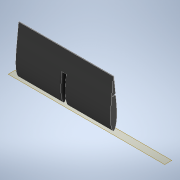
# Autodesk Inventor part: IISRD_Horizontal_tail_Control_surface
Saved by Autodesk Inventor 2021 (Build 250183000, 183)
## iProperties
Created: 2020-10-19
Part Number: IISRD_Horizontal_tail_Control_surface
Material: EPP Foam
Document SubType Name: Modeling
Designer: Kanenas
Mass: 7.28313 g
Surface Area: 775.374 cm^2
Volume: 364.157 cm^3
Density: 0.02 g/cm^3
Appearance: Generic
Author: Kanenas
Autodesk Inventor part; units mm, degrees
ref_plane "YZ Plane" through (0, 0, 0) normal (1, 0, 0) x (0, 1, 0)
sketch "Sketch1" plane through (0, 0, 0) normal (1, 0, 0) x (0, 1, 0)
  spline S0 degree 5 poles (140, 0) (140, 0.008) (139.6909, 0.023) (138.2456, 0.0648) (138.0851, 0.2448) (134.3445, 0.4509) (132.587, 0.7525) (128.0169, 1.03) (124.0758, 1.4239) (118.6617, 1.8648) (113.1342, 2.4056) (106.871, 3.0117) (100.3305, 3.6855) (93.4209, 4.4087) (86.3255, 5.1563) (79.0958, 5.9053) (71.8372, 6.629) (64.6288, 7.2884) (57.549, 7.8613) (50.671, 8.3132) (44.0585, 8.6184) (37.7676, 8.751) (31.8409, 8.7076) (26.336, 8.4735) (21.2773, 8.0467) (16.7064, 7.4272) (12.6313, 6.6359) (9.1041, 5.7147) (6.0909, 4.6974) (3.705, 3.6163) (1.758, 2.4782) (0.495, 1.2916) (-0.4137, 0) (0.495, -1.2916) (1.758, -2.4782) (3.705, -3.6163) (6.0909, -4.6974) (9.1041, -5.7147) (12.6313, -6.6359) (16.7064, -7.4272) (21.2773, -8.0467) (26.336, -8.4735) (31.8409, -8.7076) (37.7676, -8.751) (44.0585, -8.6184) (50.671, -8.3132) (57.549, -7.8613) (64.6288, -7.2884) (71.8372, -6.629) (79.0958, -5.9053) (86.3255, -5.1563) (93.4209, -4.4087) (100.3305, -3.6855) (106.871, -3.0117) (113.1342, -2.4056) (118.6617, -1.8648) (124.0758, -1.4239) (128.0169, -1.03) (132.587, -0.7525) (134.3445, -0.4509) (138.0851, -0.2448) (138.2456, -0.0648) (139.6909, -0.023) (140, -0.008) (140, 0) knots 0 0 0 0 0 0 0.009495 0.017637 0.028865 0.042353 0.057559 0.074188 0.092027 0.110874 0.13054 0.150849 0.171639 0.192755 0.214053 0.235397 0.256657 0.277714 0.298457 0.318784 0.338597 0.357809 0.37634 0.394116 0.411062 0.427101 0.442142 0.456085 0.468809 0.480163 0.490364 0.5 0.509636 0.519837 0.531191 0.543915 0.557858 0.572899 0.588938 0.605884 0.62366 0.642191 0.661403 0.681216 0.701543 0.722286 0.743343 0.764603 0.785947 0.807245 0.828361 0.849151 0.86946 0.889126 0.907973 0.925812 0.942441 0.957647 0.971135 0.982363 0.990505 1 1 1 1 1 1
  line L0 (130, 16.3724) -> (164.1986, 16.3724)
  line L1 (164.1986, 16.3724) -> (164.1986, -9.4783)
  line L2 (164.1986, -9.4783) -> (130, -9.4783)
  line L3 (130, -9.4783) -> (130, 16.3724)
  line L4 (37.4346, 8.7094) -> (37.4346, -8.7094) construction
  line L5 (20.881, 23.052) -> (20.881, -17.073) construction
  line L6 (57.3608, 24.3842) -> (57.3608, -18.5196) construction
  line L7 (20.881, -17.073) -> (57.3608, -17.073) construction
  line L8 (39.1209, -17.073) -> (39.1209, 13.7303) construction
  point P0 (138.0834, 0.1512)
  point P1 (135.8252, 0.3794)
  point P2 (132.797, 0.6664)
  point P3 (129.0044, 0.9884)
  point P4 (124.4796, 1.3706)
  point P5 (119.294, 1.8284)
  point P6 (113.526, 2.3674)
  point P7 (107.2624, 2.982)
  point P8 (100.5956, 3.661)
  point P9 (93.6194, 4.389)
  point P10 (86.4304, 5.1422)
  point P11 (79.1224, 5.8954)
  point P12 (71.785, 6.6192)
  point P13 (64.505, 7.28)
  point P14 (57.3608, 7.8484)
  point P15 (50.4266, 8.2936)
  point P16 (43.7668, 8.5876)
  point P17 (31.479, 8.6478)
  point P18 (25.9504, 8.393)
  point P19 (20.881, 7.9408)
  point P20 (16.2974, 7.2954)
  point P21 (12.222, 6.4778)
  point P22 (8.6772, 5.5216)
  point P23 (5.6966, 4.4618)
  point P24 (3.3082, 3.332)
  point P25 (1.533, 2.17)
  point P26 (0.4018, 1.0262)
  point P27 (0, 0)
  point P28 (0.4018, -1.0262)
  point P29 (1.533, -2.17)
  point P30 (3.3082, -3.332)
  point P31 (5.6966, -4.4618)
  point P32 (8.6772, -5.5216)
  point P33 (12.222, -6.4778)
  point P34 (16.2974, -7.2954)
  point P35 (20.881, -7.9408)
  point P36 (25.9504, -8.393)
  point P37 (31.479, -8.6478)
  point P38 (43.7668, -8.5876)
  point P39 (50.4266, -8.2936)
  point P40 (57.3608, -7.8484)
  point P41 (64.505, -7.28)
  point P42 (71.785, -6.6192)
  point P43 (79.1224, -5.8954)
  point P44 (86.4304, -5.1422)
  point P45 (93.6194, -4.389)
  point P46 (100.5956, -3.661)
  point P47 (107.2624, -2.982)
  point P48 (113.526, -2.3674)
  point P49 (119.294, -1.8284)
  point P50 (124.4796, -1.3706)
  point P51 (129.0044, -0.9884)
  point P52 (132.797, -0.6664)
  point P53 (135.8252, -0.3794)
  point P54 (138.0834, -0.1512)
  point P55 (139.5086, -0.0294)
  point P56 (130, -0.9104)
  point P57 (130, 0.9104)
  dimension "d9" = 130
  dimension "d72" = 17.4188
  dimension "d74" = 15.8816
  dimension "d75" = 15.6968
  dimension "d76" = 36.4798
  dimension "d77" = 39.1209
  dimension "d78" = 20.881
  constraints: 18 end point, 3 perpendicular, 3 vertical, 2 parallel, 1 horizontal, 1 midpoint, 1 point on line, 120 other
  measures "d9" distance from line of L3 point (0, 0)
  measures "d72" distance of L4.start L4.end
  measures "d74" distance of point (20.881, -7.941) point (20.881, 7.941)
  measures "d75" distance of point (57.361, -7.848) point (57.361, 7.848)
  measures "d76" horizontal distance of point (57.361, 7.848) point (20.881, 7.941)
  measures "d77" distance from line of point (0, 0) L8
  measures "d78" distance from line of point (0, 0) L5
extrude "Extrusion1" add sketch "Sketch1" along normal mid plane 260 contours L3 S0 picked at (63.1596, 2.072)
sketch "Sketch3" plane through (0, 0, 0) normal (0, 0, 1) x (1, 0, 0)
  line L0 (-130, 130) -> (130, 130) projected
  line L1 (0, 130) -> (0, 0)
  line L2 (260, 67.75) -> (260, 62.25) projected
  line L3 (104, 130) -> (260, 130)
  line L4 (260, 130) -> (260, 74.8457)
  line L5 (260, 74.8457) -> (104, 74.8457)
  line L6 (104, 74.8457) -> (104, 130)
  dimension "d11" = 260
  dimension "d12" = 183.8478
  dimension "d13" = 55.1543
  dimension "d14" = 156
  constraints: 10 end point, 2 parallel, 1 horizontal, 1 perpendicular, 1 point on line
  measures "d11" distance between parallel lines of L1 L2
  measures "d12" distance of L0.start L1.end
  measures "d13" distance of L5.end L3.start
  measures "d14" distance of L4.end L5.end
sketch "Sketch4" plane through (130, 0, 0) normal (1, 0, 0) x (0, 0, -1)
  line L0 (-5.3951, 84) -> (5.3822, 84)
  line L1 (-3.8951, 84) -> (9.1611, 87.4984)
  line L2 (-3.8951, 84) -> (8.5685, 80.6604)
  line L3 (7.1415, 86.9572) -> (7.696, 80.8942)
  point P0 (0, 0)
  dimension "d17" = 84
  dimension "d18" = 1.5
  dimension "d19" = 15
  dimension "d20" = 15
  constraints: 8 end point, 2 point on line, 1 horizontal, 1 other
  measures "d17" vertical distance of point (0, 0) L1.start
  measures "d18" distance of L1.start L0.start
  measures "d19" angle of L1 L0
  measures "d20" angle of L0 L2
extrude "Extrusion3" cut sketch "Sketch4" against normal through all
ref_plane "Work Plane3" through (0, 36.3757, 8.7122) normal (0, 0, 1) x (1, 0, 0)
sketch "Sketch11" plane through (0, 36.3757, 8.7122) normal (0, 0, 1) x (1, 0, 0)
  line L0 (-130, 93.6243) -> (-130, 93.6243) projected
  line L1 (130, 93.6243) -> (130, -36.3757) projected
  line L2 (130, 93.6243) -> (-130, 93.6243) projected
  line L3 (-6, 39.6243) -> (6, 39.6243)
  line L4 (6, 39.6243) -> (6, -36.3757)
  line L5 (6, -36.3757) -> (-6, -36.3757)
  line L6 (-6, -36.3757) -> (-6, 39.6243)
  line L7 (0, 39.6243) -> (0, -36.3757) construction
  line L8 (-130, -36.3757) -> (130, -36.3757) construction
  line L9 (130, 47.6243) -> (-130, 47.6243) projected
  point P0 (-130, 45.0643)
  point P1 (130, 45.0643)
  dimension "d61" = 260
  dimension "d62" = 12
  dimension "d63" = 130
  dimension "d65" = 130
  dimension "d70" = 8
  constraints: 12 end point, 2 horizontal, 2 midpoint, 2 parallel, 1 collinear, 1 perpendicular
  measures "d61" distance between parallel lines of L1 L0
  measures "d62" distance of L3.start L3.end
  measures "d63" distance between parallel lines of L0 L7
  measures "d65" distance of L1.start L1.end
  measures "d70" distance between parallel lines of L9 L3
extrude "Extrusion8" cut sketch "Sketch11" against normal through all
ref_plane "Work Plane4" through (0, 36.3757, -8.7122) normal (0, 0, -1) x (-1, 0, 0)
sketch "Sketch12" plane through (0, 36.3757, -8.7122) normal (0, 0, -1) x (-1, 0, 0)
  line L0 (30, 24.6243) -> (38.6, 24.6243)
  line L1 (38.6, 24.6243) -> (38.6, -3.3757)
  line L2 (38.6, -3.3757) -> (30, -3.3757)
  line L3 (30, -3.3757) -> (30, 24.6243)
  point P0 (0, -36.3757)
  dimension "d79" = 33
  dimension "d80" = 8.6
  dimension "d81" = 28
  dimension "d82" = 30
  constraints: 8 end point, 2 parallel, 1 horizontal, 1 perpendicular
  measures "d79" distance from line of L2 point (0, -36.376)
  measures "d80" distance between parallel lines of L3 L1
  measures "d81" distance between parallel lines of L2 L0
  measures "d82" distance from line of L3 point (0, -36.376)
extrude "Extrusion9" cut sketch "Sketch12" against normal blind 2
sketch "Sketch14" plane through (0, 36.3757, -8.7122) normal (0, 0, -1) x (-1, 0, 0)
  line L0 (25, 88.6243) -> (26, 88.6243)
  line L1 (26, 88.6243) -> (26, 68.6243)
  line L2 (26, 68.6243) -> (25, 68.6243)
  line L3 (25, 68.6243) -> (25, 88.6243)
  point P0 (0, -36.3757)
  dimension "d85" = 20
  dimension "d86" = 1
  dimension "d87" = 25
  dimension "d88" = 105
  constraints: 8 end point, 2 parallel, 1 horizontal, 1 perpendicular
  measures "d85" distance of L2.end L0.start
  measures "d86" distance of L1.end L2.end
  measures "d87" distance from line of L3 point (0, -36.376)
  measures "d88" distance from line of L2 point (0, -36.376)
extrude "Extrusion10" cut sketch "Sketch14" against normal blind 8
equation "\"d13\" = 0.3 * d12"
equation "\"d14\" = 0.6 * d11"
equation "\"d63\" = 0.5 * d61"
body "Solid1"
